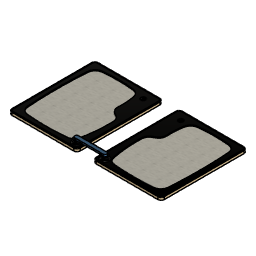
Maos IEB v4 (Autodesk Fusion 360 design; units mm, degrees)
Autodesk Fusion 360 part; units mm, degrees
sketch "Sketch1" plane through (0, 0, 0) normal (0, 0, 1) x (1, 0, 0)
  line L0 (-228.8074, -5) -> (-35, -5)
  line L1 (-25, -15) -> (-25, -265)
  line L2 (-35, -275) -> (-228.8074, -275)
  line L3 (-238.8074, -265) -> (-238.8074, -15)
  arc A0 (-218.8074, -25) -> (-218.8074, -255) centre (1101.1926, -140) ccw
  arc A1 (-83.5994, -25) -> (-218.8074, -25) centre (-151.2034, -479.5304) ccw
  arc A2 (-78.8074, -116.436) -> (-83.5994, -25) centre (-288.0073, -81.5561) ccw
  arc A3 (-45, -125.4947) -> (-78.8074, -116.436) centre (-81.4607, -193.9531) ccw
  arc A4 (-218.8074, -255) -> (-56.3302, -255) centre (-137.5688, 402.4707) ccw
  arc A5 (-56.3302, -255) -> (-45, -125.4947) centre (-469.0669, -153.6419) ccw
  line L4 (-218.8074, -255) -> (-218.8074, -25) construction
  line L5 (-218.8074, -25) -> (-83.5994, -25) construction
  line L6 (-78.8074, -116.436) -> (-83.5994, -25) construction
  line L7 (-78.8074, -116.436) -> (-45, -125.4947) construction
  line L8 (-45, -125.4947) -> (-56.3302, -255) construction
  line L9 (-56.3302, -255) -> (-218.8074, -255) construction
  line L10 (-223.8074, -140) -> (-218.8074, -140) construction
  line L11 (-151.2034, -20) -> (-151.2034, -25) construction
  line L12 (-76.2102, -70.4563) -> (-81.2034, -70.718) construction
  line L13 (-50.6651, -190.2473) -> (-45.6841, -190.6831) construction
  line L14 (-137.5688, -255) -> (-137.5688, -260) construction
  line L15 (-61.3861, -119.0335) -> (-61.9037, -120.9654) construction
  arc A6 (-228.8074, -5) -> (-238.8074, -15) centre (-228.8074, -15) ccw
  arc A7 (-25, -15) -> (-35, -5) centre (-35, -15) ccw
  arc A8 (-35, -275) -> (-25, -265) centre (-35, -265) ccw
  arc A9 (-238.8074, -265) -> (-228.8074, -275) centre (-228.8074, -265) ccw
  line L16 (0, 0) -> (0, -43.4181) construction
  arc A10 (-28, -15) -> (-35, -8) centre (-35, -15) ccw
  line L17 (-228.8074, -8) -> (-35, -8)
  arc A11 (-228.8074, -8) -> (-235.8074, -15) centre (-228.8074, -15) ccw
  line L18 (-235.8074, -265) -> (-235.8074, -15)
  arc A12 (-235.8074, -265) -> (-228.8074, -272) centre (-228.8074, -265) ccw
  line L19 (-35, -272) -> (-228.8074, -272)
  arc A13 (-35, -272) -> (-28, -265) centre (-35, -265) ccw
  line L20 (-28, -15) -> (-28, -265)
  line L21 (-235.5074, -265) -> (-235.5074, -15)
  arc A14 (-228.8074, -8.3) -> (-235.5074, -15) centre (-228.8074, -15) ccw
  line L22 (-228.8074, -8.3) -> (-35, -8.3)
  arc A15 (-28.3, -15) -> (-35, -8.3) centre (-35, -15) ccw
  line L23 (-28.3, -15) -> (-28.3, -265)
  arc A16 (-35, -271.7) -> (-28.3, -265) centre (-35, -265) ccw
  line L24 (-35, -271.7) -> (-228.8074, -271.7)
  arc A17 (-235.5074, -265) -> (-228.8074, -271.7) centre (-228.8074, -265) ccw
  dimension "d1" = 95
  dimension "d2" = 100
  dimension "d3" = 93
  dimension "d4" = 20
  dimension "d5" = 20
  dimension "d6" = 5
  dimension "d7" = 2
  dimension "d8" = 5
  dimension "d9" = 20
  dimension "d10" = 20
  dimension "d11" = 10
  dimension "d12" = 3
  dimension "d13" = -3.3
  dimension "d25" = 25
  dimension "d26" = 5
  dimension "d61" = 140
  dimension "d62" = 230
  dimension "d63" = 130
  dimension "d64" = 35
  constraint horizontal L0
  constraint vertical L1
  constraint horizontal L2
  constraint vertical L3
  constraint horizontal L9
  constraint horizontal L5
  constraint vertical L4
  constraint midpoint A0 L10.start
  constraint midpoint L4 L10.end
  constraint midpoint A1 L11.start
  constraint midpoint L5 L11.end
  constraint midpoint A2 L12.start
  constraint midpoint L6 L12.end
  constraint midpoint L8 L13.start
  constraint midpoint A5 L13.end
  constraint midpoint L9 L14.start
  constraint midpoint A4 L14.end
  constraint midpoint A3 L15.start
  constraint midpoint L7 L15.end
  constraint equal L10 L11
  constraint equal L11 L12
  constraint equal L10 L14
  constraint tangent L0 A6
  constraint tangent L3 A6
  constraint tangent L0 A7
  constraint tangent L1 A7
  constraint equal A6 A7
  constraint tangent L1 A8
  constraint tangent L2 A8
  constraint equal A6 A8
  constraint tangent L2 A9
  constraint tangent L3 A9
  constraint equal A6 A9
  constraint coincident L16.start origin
  constraint vertical L16
  measures "d1" angle of L8 L9
  measures "d2" angle of L7 L8
  measures "d3" angle of L5 L6
  measures "d4" distance of L0 L5
  measures "d5" distance of L3 L4
  measures "d6" distance of L10.start L10.end
  measures "d7" distance of L15.start L15.end
  measures "d8" distance of L13.start L13.end
  measures "d9" distance of L2 L9
  measures "d10" distance of L1 A3.start
  measures "d11" radius of A6
  measures "d25" distance of L1 L16
  measures "d26" distance of L16.start L0
  measures "d61" distance of A2.start L4
  measures "d62" distance of L5 L9
  measures "d63" distance of A3.start A4.end
  measures "d64" distance of A2.start A3.start
extrude "Extrude1" add sketch "Sketch1" against normal blind 3 contours L0 L1 L2 L3 A6 A7 A8 A9 | A0 A1 A2 A3 A4 A5 | A10 L17 A11 L18 A12 L19 A13 L20 | L21 A14 L22 A15 L23 A16 L24 A17 makes body 1
extrude "Extrude2" add sketch "Sketch1" along normal blind 5 contours L0 L1 L2 L3 A6 A7 A8 A9 bodies 1
extrude "Extrude1'" add sketch "Sketch1" along normal blind 3 separate body contours L21 A14 L22 A15 L23 A16 L24 A17 makes body 2 in component "Component"
fillet "Fillet1" radius 25 6 edges at (-218.8074, -25, 1.5) (-83.5994, -25, 1.5) (-78.8074, -116.436, 1.5) (-45, -125.4947, 1.5) (-56.3302, -255, 1.5) (-218.8074, -255, 1.5) on bodies 2 in component "Component"
sketch "Sketch2" plane through (0, 0, 3) normal (0, 0, 1) x (-1, 0, 0)
  line L0 (28.3, 265) -> (28.3, 15)
  line L1 (35, 8.3) -> (228.8074, 8.3)
  line L2 (235.5074, 15) -> (235.5074, 265)
  line L3 (228.8074, 271.7) -> (35, 271.7)
  arc A0 (76.3086, 94.3954) -> (60.2868, 119.2587) centre (51.3544, 95.9089) ccw
  arc A1 (44.2286, 141.9189) -> (60.2868, 119.2587) centre (69.2191, 142.6085) ccw
  arc A2 (52.3227, 237.0041) -> (44.2286, 141.9189) centre (469.0669, 153.6419) ccw
  arc A3 (74.4553, 256.9867) -> (52.3227, 237.0041) centre (76.837, 232.1004) ccw
  arc A4 (197.7951, 257.2567) -> (74.4553, 256.9867) centre (137.5688, -402.4707) ccw
  arc A5 (220.4592, 234.1364) -> (197.7951, 257.2567) centre (195.5223, 232.3602) ccw
  arc A6 (220.4318, 45.4799) -> (220.4592, 234.1364) centre (-1101.1926, 140) ccw
  arc A7 (198.0437, 22.3935) -> (220.4318, 45.4799) centre (195.4955, 47.2633) ccw
  arc A8 (101.3189, 22.7156) -> (198.0437, 22.3935) centre (151.2034, 479.5304) ccw
  arc A9 (79.4488, 43.0261) -> (101.3189, 22.7156) centre (104.0328, 47.5679) ccw
  arc A10 (76.3086, 94.3954) -> (79.4488, 43.0261) centre (288.0073, 81.5561) ccw
  circle A11 centre (59, 33.3) radius 7.5
  circle A12 centre (-59, 33.3) radius 7.5
  line L4 (-59, 33.3) -> (59, 33.3) construction
  line L5 (0, 33.3) -> (0, 0)
  line L6 (61.3094, 29.3) -> (63.6188, 33.3)
  line L7 (63.6188, 33.3) -> (61.3094, 37.3)
  line L8 (61.3094, 37.3) -> (56.6906, 37.3)
  line L9 (56.6906, 37.3) -> (54.3812, 33.3)
  line L10 (54.3812, 33.3) -> (56.6906, 29.3)
  line L11 (56.6906, 29.3) -> (61.3094, 29.3)
  circle A13 centre (44.3, 256.7) radius 6
  circle A14 centre (-63.1507, 257.4382) radius 46.1789
  circle A15 centre (44.3, 256.7) radius 10
  line L12 (0, 33.3) -> (0, 410.3453)
  circle A16 centre (44.3, 256.7) radius 5.8
  arc A17 (228.8074, 8.3) -> (235.5074, 15) centre (228.8074, 15) ccw
  arc A18 (235.5074, 265) -> (228.8074, 271.7) centre (228.8074, 265) ccw
  arc A19 (35, 271.7) -> (28.3, 265) centre (35, 265) ccw
  arc A20 (28.3, 15) -> (35, 8.3) centre (35, 15) ccw
  point P0 (59, 33.3)
  dimension "d29" = 25
  dimension "d30" = 118
  dimension "d31" = 15
  dimension "d35" = 8
  dimension "d38" = 4
  dimension "d39" = 12
  dimension "d44" = 16
  dimension "d45" = 0.2
  dimension "d65" = 15
  constraint coincident A12.centre L4.start
  constraint coincident P0 A11.centre
  constraint horizontal L4
  constraint equal A11 A12
  constraint midpoint L4 L5.start
  constraint perpendicular L4 L5
  constraint coincident L5.end origin
  constraint concentric A13 A15
  constraint perpendicular L4 L12
  constraint concentric A15 A16
  constraint horizontal L11
  measures "d29" distance of L1 L4
  measures "d30" distance of A12.centre P0
  measures "d31" diameter of A11
  measures "d35" distance of L7 L10
  measures "d38" distance of A13 A15
  measures "d39" diameter of A13
  measures "d44" distance of L0 A13.centre
  measures "d45" distance of A13 A16
  measures "d65" distance of L3 A13.centre
extrude "Extrude2'" cut sketch "Sketch2" against normal blind 20 contours A11 | L6 L7 L8 L9 L10 L11 bodies 2 in component "Component"
extrude "Extrude3" cut sketch "Sketch2" against normal blind 8 contours L6 L7 L8 L9 L10 L11 bodies 1
extrude "Extrude3'" add sketch "Sketch2" along normal blind 10 contours A15 bodies 2 in component "Component"
fillet "Fillet2" radius 4 1 edges at (-34.9767, -260.3162, 3) on bodies 2 in component "Component"
sketch "Sketch3" plane through (0, 0, 13) normal (0, 0, 1) x (-1, 0, 0)
  circle A0 centre (44.3, 256.7) radius 6
  circle A1 centre (44.3, 256.7) radius 10
  line L0 (0, 0) -> (0, -76.6678)
  line L1 (0, -76.6678) -> (0, 297.2205)
  circle A2 centre (44.3, 256.7) radius 5.8
  line L2 (44.4656, 250.9024) -> (0, 250.9024)
  line L3 (44.3, 262.5) -> (0, 262.5)
  dimension "d46" = -0.2
  constraint coincident L0.start origin
  constraint vertical L0
  constraint parallel L0 L1
  constraint coincident A2 L2.start
  constraint coincident L1 L2.end
  constraint perpendicular L1 L2
  constraint coincident A2 L3.start
  constraint coincident L1 L3.end
  constraint tangent A2 L3
  constraint perpendicular L1 L3
extrude "Extrude4" add sketch "Sketch3" against normal blind 10 from surface at 1 separate body contours A2 L2 picked at (45.9803, 258.1985) makes body 3
extrude "Extrude5" add sketch "Sketch3" along normal blind 5 from surface at 1 contours A0 A2 L2 L3 | A0 A1 L2 L3 | A2 L2 | A1 L1 L2 L3 picked at (39.9251, 252.8072) picked at (35.6491, 256.7025) picked at (45.9803, 258.1985) bodies 3
mirror "Mirror2" about plane through (0, -250.9024, 14) normal (1, 0, 0) of bodies 3 merged
mirror "Mirror3" about plane through (0, 0, 0) normal (1, 0, 0) of bodies 1 makes body 4
mirror "Mirror1" about plane through (0, 0, 0) normal (1, 0, 0) of bodies 2 makes body 5 in component "Component"
move_body "Move1" bodies 3 to x (1, 0, 0) y (0, 1, 0) z (0, 0, 1) at (0, 0, 3)
move_body "Move1'" bodies 2 5 to x (1, 0, 0) y (0, 1, 0) z (0, 0, 1) at (0, 0, 3) in component "Component"
extrude "Extrude6" add 2 faces at (-108.3723, -189.1, 0) (108.3723, -189.1, 0) along direction (0, 0, 1) blind 3 separate body on bodies 1 4 makes body 6 at (-108.3723, -189.1, 0) makes body 7 at (108.3723, -189.1, 0)
component "Component" placed x (1, 0, 0) y (0, 1, 0) z (0, 0, 1) at (0, 0, 0)
